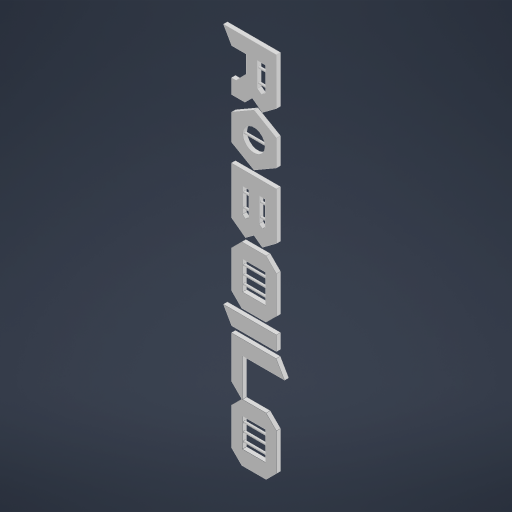
# Autodesk Inventor part: roboilo
Saved by Autodesk Inventor 2024 (Build 280153000, 153)
## iProperties
Created: 2024-06-09
Part Number: roboilo
Material: Generic
Document SubType Name: Modeling
Designer: mateu
Density: 1 g/cm^3
Appearance: Default
Author: mateu
Autodesk Inventor part; units mm, degrees
ref_plane "YZ Plane" through (0, 0, 0) normal (1, 0, 0) x (0, 1, 0)
ref_plane "XZ Plane" through (0, 0, 0) normal (0, 1, 0) x (-1, 0, 0)
ref_plane "XY Plane" through (0, 0, 0) normal (0, 0, 1) x (1, 0, 0)
sketch "Sketch1" plane through (0, 0, 0) normal (0, 0, 1) x (1, 0, 0)
  line L0 (13.187, 45.2611) -> (13.187, 52.8058) construction
  line L1 (11.8207, 44.2163) -> (13.187, 45.2611) construction
  line L2 (10.3841, 45.2712) -> (11.8207, 44.2163) construction
  line L3 (10.3841, 52.8058) -> (10.3841, 45.2712) construction
  line L4 (13.187, 52.8058) -> (10.3841, 52.8058) construction
  line L5 (3.0806, 40.1778) -> (3.0806, 44.1058) construction
  line L6 (6.8077, 40.1778) -> (3.0806, 40.1778) construction
  line L7 (9.0681, 42.4281) -> (6.8077, 40.1778) construction
  line L8 (12.0919, 40.1778) -> (9.0681, 42.4281) construction
  line L9 (16.0802, 43.1414) -> (12.0919, 40.1778) construction
  line L10 (16.0802, 56.7338) -> (16.0802, 43.1414) construction
  line L11 (0.8302, 56.7338) -> (16.0802, 56.7338) construction
  line L12 (3.0806, 52.8058) -> (0.8302, 56.7338) construction
  line L13 (7.4305, 52.8058) -> (3.0806, 52.8058) construction
  line L14 (7.4305, 47.3013) -> (7.4305, 52.8058) construction
  line L15 (4.3156, 44.1058) -> (7.4305, 47.3013) construction
  line L16 (3.0806, 44.1058) -> (4.3156, 44.1058) construction
  line L17 (3.0806, 27.8164) -> (3.0806, 35.3218) construction
  line L18 (9.5804, 24.0637) -> (3.0806, 27.8164) construction
  line L19 (16.0802, 27.8164) -> (9.5804, 24.0637) construction
  line L20 (16.0802, 35.3218) -> (16.0802, 27.8164) construction
  line L21 (9.5804, 39.0745) -> (16.0802, 35.3218) construction
  line L22 (3.0806, 35.3218) -> (9.5804, 39.0745) construction
  circle A0 centre (9.5804, 31.5691) radius 3.5 construction
  line L23 (13.1669, 10.6183) -> (13.1669, 18.163) construction
  line L24 (12.0819, 9.664) -> (13.1669, 10.6183) construction
  line L25 (10.8965, 10.6183) -> (12.0819, 9.664) construction
  line L26 (10.8965, 18.163) -> (10.8965, 10.6183) construction
  line L27 (13.1669, 18.163) -> (10.8965, 18.163) construction
  line L28 (8.2443, 10.6183) -> (8.2443, 18.163) construction
  line L29 (7.0588, 9.664) -> (8.2443, 10.6183) construction
  line L30 (5.9739, 10.6183) -> (7.0588, 9.664) construction
  line L31 (5.9739, 18.163) -> (5.9739, 10.6183) construction
  line L32 (8.2443, 18.163) -> (5.9739, 18.163) construction
  line L33 (7.0588, 5.3642) -> (3.0605, 8.3178) construction
  line L34 (9.5704, 7.2127) -> (7.0588, 5.3642) construction
  line L35 (12.0819, 5.3642) -> (9.5704, 7.2127) construction
  line L36 (16.0802, 8.3178) -> (12.0819, 5.3642) construction
  line L37 (16.0802, 22.091) -> (16.0802, 8.3178) construction
  line L38 (3.0605, 22.091) -> (16.0802, 22.091) construction
  line L39 (3.0605, 8.3178) -> (3.0605, 22.091) construction
  line L40 (13.187, -9.5241) -> (13.187, -0.6233) construction
  line L41 (5.9739, -9.5241) -> (13.187, -9.5241) construction
  line L42 (5.9739, -0.6233) -> (5.9739, -9.5241) construction
  line L43 (13.187, -0.6233) -> (5.9739, -0.6233) construction
  line L44 (6.0341, -13.4521) -> (3.0806, -10.4986) construction
  line L45 (13.1267, -13.4521) -> (6.0341, -13.4521) construction
  line L46 (16.0802, -10.4986) -> (13.1267, -13.4521) construction
  line L47 (16.0802, 0.3512) -> (16.0802, -10.4986) construction
  line L48 (13.1267, 3.3048) -> (16.0802, 0.3512) construction
  line L49 (6.0341, 3.3048) -> (13.1267, 3.3048) construction
  line L50 (3.0806, 0.3512) -> (6.0341, 3.3048) construction
  line L51 (3.0806, -10.4986) -> (3.0806, 0.3512) construction
  line L52 (3.0605, -19.4798) -> (0.8302, -15.5518) construction
  line L53 (16.0802, -19.4798) -> (3.0605, -19.4798) construction
  line L54 (16.0802, -15.5518) -> (16.0802, -19.4798) construction
  line L55 (0.8302, -15.5518) -> (16.0802, -15.5518) construction
  line L56 (5.9739, -36.8094) -> (3.0605, -33.896) construction
  line L57 (5.9739, -25.6381) -> (5.9739, -36.8094) construction
  line L58 (18.3607, -25.6381) -> (5.9739, -25.6381) construction
  line L59 (16.0903, -21.7101) -> (18.3607, -25.6381) construction
  line L60 (3.0605, -21.7101) -> (16.0903, -21.7101) construction
  line L61 (3.0605, -33.896) -> (3.0605, -21.7101) construction
  line L62 (13.187, -50.0803) -> (13.187, -41.1794) construction
  line L63 (5.9739, -50.0803) -> (13.187, -50.0803) construction
  line L64 (5.9739, -41.1794) -> (5.9739, -50.0803) construction
  line L65 (13.187, -41.1794) -> (5.9739, -41.1794) construction
  line L66 (6.0341, -54.0083) -> (3.0806, -51.0548) construction
  line L67 (13.1267, -54.0083) -> (6.0341, -54.0083) construction
  line L68 (16.0802, -51.0548) -> (13.1267, -54.0083) construction
  line L69 (16.0802, -40.2049) -> (16.0802, -51.0548) construction
  line L70 (13.1267, -37.2514) -> (16.0802, -40.2049) construction
  line L71 (6.0341, -37.2514) -> (13.1267, -37.2514) construction
  line L72 (3.0806, -40.2049) -> (6.0341, -37.2514) construction
  line L73 (3.0806, -51.0548) -> (3.0806, -40.2049) construction
  line L74 (7.2305, 52.6058) -> (2.9647, 52.6058)
  line L75 (2.9647, 52.6058) -> (0.4852, 56.9338)
  line L76 (0.4852, 56.9338) -> (16.2802, 56.9338)
  line L77 (16.2802, 56.9338) -> (16.2802, 43.0408)
  line L78 (16.2802, 43.0408) -> (12.0919, 39.9286)
  line L79 (12.0919, 39.9286) -> (9.087, 42.1647)
  line L80 (9.087, 42.1647) -> (6.8903, 39.9778)
  line L81 (6.8903, 39.9778) -> (2.8806, 39.9778)
  line L82 (2.8806, 39.9778) -> (2.8806, 44.3058)
  line L83 (2.8806, 44.3058) -> (4.2313, 44.3058)
  line L84 (4.2313, 44.3058) -> (7.2305, 47.3827)
  line L85 (7.2305, 47.3827) -> (7.2305, 52.6058)
  line L86 (11.8183, 44.4662) -> (12.987, 45.36)
  line L87 (12.987, 45.36) -> (12.987, 52.6058)
  line L88 (12.987, 52.6058) -> (10.5841, 52.6058)
  line L89 (10.5841, 52.6058) -> (10.5841, 45.3724)
  line L90 (10.5841, 45.3724) -> (11.8183, 44.4662)
  circle A1 centre (9.5804, 31.5691) radius 3.3
  line L91 (9.5804, 39.3054) -> (16.2802, 35.4373)
  line L92 (16.2802, 35.4373) -> (16.2802, 27.7009)
  line L93 (16.2802, 27.7009) -> (9.5804, 23.8328)
  line L94 (9.5804, 23.8328) -> (2.8806, 27.7009)
  line L95 (2.8806, 27.7009) -> (2.8806, 35.4373)
  line L96 (2.8806, 35.4373) -> (9.5804, 39.3054)
  line L97 (16.2802, 22.291) -> (16.2802, 8.2169)
  line L98 (16.2802, 8.2169) -> (12.0821, 5.1157)
  line L99 (12.0821, 5.1157) -> (9.5704, 6.9644)
  line L100 (9.5704, 6.9644) -> (7.0586, 5.1157)
  line L101 (7.0586, 5.1157) -> (2.8605, 8.2169)
  line L102 (2.8605, 8.2169) -> (2.8605, 22.291)
  line L103 (2.8605, 22.291) -> (16.2802, 22.291)
  line L104 (8.0443, 17.963) -> (8.0443, 10.7141)
  line L105 (8.0443, 10.7141) -> (7.0645, 9.9253)
  line L106 (7.0645, 9.9253) -> (6.1739, 10.7088)
  line L107 (6.1739, 10.7088) -> (6.1739, 17.963)
  line L108 (6.1739, 17.963) -> (8.0443, 17.963)
  line L109 (11.0965, 10.7141) -> (12.0762, 9.9253)
  line L110 (12.0762, 9.9253) -> (12.9669, 10.7088)
  line L111 (12.9669, 10.7088) -> (12.9669, 17.963)
  line L112 (12.9669, 17.963) -> (11.0965, 17.963)
  line L113 (11.0965, 17.963) -> (11.0965, 10.7141)
  line L114 (13.2095, 3.5048) -> (16.2802, 0.4341)
  line L115 (16.2802, 0.4341) -> (16.2802, -10.5814)
  line L116 (16.2802, -10.5814) -> (13.2095, -13.6521)
  line L117 (13.2095, -13.6521) -> (5.9513, -13.6521)
  line L118 (5.9513, -13.6521) -> (2.8806, -10.5814)
  line L119 (2.8806, -10.5814) -> (2.8806, 0.4341)
  line L120 (2.8806, 0.4341) -> (5.9513, 3.5048)
  line L121 (5.9513, 3.5048) -> (13.2095, 3.5048)
  line L122 (6.1739, -0.8233) -> (6.1739, -9.3241)
  line L123 (6.1739, -9.3241) -> (12.987, -9.3241)
  line L124 (12.987, -9.3241) -> (12.987, -0.8233)
  line L125 (12.987, -0.8233) -> (6.1739, -0.8233)
  line L126 (16.2802, -15.3518) -> (16.2802, -19.6798)
  line L127 (16.2802, -19.6798) -> (2.9441, -19.6798)
  line L128 (2.9441, -19.6798) -> (0.4867, -15.3518)
  line L129 (0.4867, -15.3518) -> (16.2802, -15.3518)
  line L130 (6.1739, -37.2922) -> (2.8605, -33.9788)
  line L131 (2.8605, -33.9788) -> (2.8605, -21.5101)
  line L132 (2.8605, -21.5101) -> (16.2057, -21.5101)
  line L133 (16.2057, -21.5101) -> (18.7073, -25.8381)
  line L134 (18.7073, -25.8381) -> (6.1739, -25.8381)
  line L135 (6.1739, -25.8381) -> (6.1739, -37.2922)
  line L136 (13.2095, -37.0514) -> (16.2802, -40.1221)
  line L137 (16.2802, -40.1221) -> (16.2802, -51.1376)
  line L138 (16.2802, -51.1376) -> (13.2095, -54.2083)
  line L139 (13.2095, -54.2083) -> (5.9513, -54.2083)
  line L140 (5.9513, -54.2083) -> (2.8806, -51.1376)
  line L141 (2.8806, -51.1376) -> (2.8806, -40.1221)
  line L142 (2.8806, -40.1221) -> (5.9513, -37.0514)
  line L143 (5.9513, -37.0514) -> (13.2095, -37.0514)
  line L144 (6.1739, -41.3794) -> (6.1739, -49.8803)
  line L145 (6.1739, -49.8803) -> (12.987, -49.8803)
  line L146 (12.987, -49.8803) -> (12.987, -41.3794)
  line L147 (12.987, -41.3794) -> (6.1739, -41.3794)
  point P0 (0, 0)
  point P1 (6.1739, -37.0514)
  point P2 (5.9422, -37.0605)
extrude "Extrusion1" add sketch "Sketch1" along normal blind 1.2
sketch "Sketch2" plane through (6.1739, -9.3241, 0) normal (1, 0, 0) x (0, 0, -1)
  line L0 (0, 0) -> (0, 8.5009) projected
  line L1 (0, 8.5009) -> (-1.2, 8.5009) projected
  line L2 (-1.2, 0) -> (-1.2, 8.5009) projected
  line L3 (0, 0) -> (-1.2, 0) projected
  line L4 (-0.6, 8.5009) -> (-0.6, 0)
  line L5 (-0.6, 4.2504) -> (0, 4.2504)
  line L6 (0, 9.7582) -> (0, -1.2573) projected
  circle A0 centre (-0.6, 6.7504) radius 0.3
  circle A1 centre (-0.6, 4.2504) radius 0.3
  circle A2 centre (-0.6, 1.7504) radius 0.3
  line L7 (0, -40.5562) -> (0, -32.0553) projected
  line L8 (0, -32.0553) -> (-1.2, -32.0553) projected
  line L9 (-1.2, -40.5562) -> (-1.2, -32.0553) projected
  line L10 (0, -40.5562) -> (-1.2, -40.5562) projected
  circle A3 centre (-0.6, -33.8057) radius 0.3
  circle A4 centre (-0.6, -36.3057) radius 0.3
  circle A5 centre (-0.6, -38.8057) radius 0.3
  point P0 (0, 9.3241)
  dimension "d15" = 2.5
  dimension "d16" = 0.6
  dimension "d17" = 0.6
  dimension "d18" = 0.6
  dimension "d19" = 2.5
  dimension "d20" = 2.5
  dimension "d21" = 0.6
  dimension "d22" = 0.6
  dimension "d23" = 0.6
  constraints: 6 centre point, 6 coincident, 4 end point, 4 midpoint, 2 point on line, 1 symmetric about line, 1 other
  measures "d15" distance from line of L5 point (-0.6, 1.75)
  measures "d16" diameter of A0
  measures "d17" diameter of A1
  measures "d18" diameter of A2
  measures "d19" distance of point (-0.6, -36.306) point (-0.6, -33.806)
  measures "d20" distance of point (-0.6, -38.806) point (-0.6, -36.306)
  measures "d21" diameter of A3
  measures "d22" diameter of A4
  measures "d23" diameter of A5
extrude "Extrusion2" add sketch "Sketch2" along normal blind 9 contours A1 L4 L5 | L5 L4 A1 | A2 L4 | L4 A2 | L4 A1 | A0 L4 | L4 A0 | A3 | A4 | A5
sketch "Sketch3" plane through (10.5841, 45.3724, 0) normal (1, 0, 0) x (0, 0, -1)
  line L0 (0, 0) -> (0, 7.2333) projected
  line L1 (0, 7.2333) -> (-1.2, 7.2333) projected
  line L2 (-1.2, 0) -> (-1.2, 7.2333) projected
  line L3 (0, 0) -> (-1.2, 0) projected
  line L4 (0, -0.9062) -> (0, 0) projected
  line L5 (0, 0) -> (-1.2, 0) projected
  line L6 (-1.2, -0.9062) -> (-1.2, 0) projected
  line L7 (0, -0.9062) -> (-1.2, -0.9062) projected
  circle A0 centre (-0.6, 5.2166) radius 0.3
  circle A1 centre (-0.6, 1.2204) radius 0.3
  point P0 (0, -45.3724)
  dimension "d26" = 0.6
  dimension "d27" = 0.6
  constraints: 2 centre point
  measures "d26" diameter of A0
  measures "d27" diameter of A1
extrude "Extrusion3" add sketch "Sketch3" along normal blind 3 contours A0 | A1
sketch "Sketch4" plane through (6.1739, 10.7088, 0) normal (1, 0, 0) x (0, 0, -1)
  line L0 (0, 0) -> (0, 7.2542) projected
  line L1 (0, 7.2542) -> (-1.2, 7.2542) projected
  line L2 (-1.2, 0) -> (-1.2, 7.2542) projected
  line L3 (0, 0) -> (-1.2, 0) projected
  line L4 (0, -0.7835) -> (0, 0) projected
  line L5 (0, 0) -> (-1.2, 0) projected
  line L6 (-1.2, -0.7835) -> (-1.2, 0) projected
  line L7 (0, -0.7835) -> (-1.2, -0.7835) projected
  circle A0 centre (-0.6, 5.4648) radius 0.3
  circle A1 centre (-0.6, 1.5016) radius 0.3
  line L8 (-1.2, 17.5603) -> (-1.2, 24.1603) projected
  line L9 (0, 17.5603) -> (0, 24.1603) projected
  circle A2 centre (-0.6, 20.8603) radius 0.3
  point P0 (0, -10.7088)
  dimension "d30" = 0.6
  dimension "d31" = 0.6
  dimension "d32" = 0.6
  constraints: 3 centre point
  measures "d30" diameter of A0
  measures "d31" diameter of A1
  measures "d32" diameter of A2
extrude "Extrusion4" add sketch "Sketch4" along normal up to surface (10.1064 mm away) contours A0 | A1 | A2
body "Solid1"
